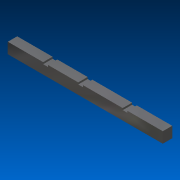
# Autodesk Inventor part: SPACER REAR B 1
Saved by Autodesk Inventor 2012 (Build 160160000, 160)
## iProperties
Created: 2012-07-06
Part Number: SPACER REAR B 1
Material: Default
Document SubType Name: Modeling
Designer: Hemant
Density: 1 g/cm^3
Author: Hemant
Autodesk Inventor part; units mm, degrees
ref_plane "YZ Plane" through (0, 0, 0) normal (1, 0, 0) x (0, 1, 0)
ref_plane "XZ Plane" through (0, 0, 0) normal (0, 1, 0) x (-1, 0, 0)
ref_plane "XY Plane" through (0, 0, 0) normal (0, 0, 1) x (1, 0, 0)
sketch "Sketch1" plane through (0, 0, 0) normal (0, 0, 1) x (1, 0, 0)
  line L0 (0, 0) -> (0, 58.2168)
  line L1 (0, 58.2168) -> (190.5, 58.2168)
  line L2 (190.5, 58.2168) -> (190.5, 48.6918)
  line L3 (190.5, 48.6918) -> (215.9, 48.6918)
  line L4 (215.9, 48.6918) -> (215.9, 58.2168)
  line L5 (215.9, 58.2168) -> (379.476, 58.2168)
  line L6 (379.476, 58.2168) -> (379.476, 48.6918)
  line L7 (379.476, 48.6918) -> (404.876, 48.6918)
  line L8 (404.876, 48.6918) -> (404.876, 58.2168)
  line L9 (404.876, 58.2168) -> (619.125, 58.2168)
  line L10 (619.125, 58.2168) -> (619.125, 48.6918)
  line L11 (619.125, 48.6918) -> (644.525, 48.6918)
  line L12 (644.525, 48.6918) -> (644.525, 58.2168)
  line L13 (644.525, 58.2168) -> (835.025, 58.2168)
  line L14 (835.025, 58.2168) -> (835.025, 0)
  line L15 (835.025, 0) -> (0, 0)
  dimension "d0" = 58.2168
  dimension "d1" = 835.025
  dimension "d2" = 190.5
  dimension "d3" = 25.4
  dimension "d4" = 25.4
  dimension "d5" = 25.4
  dimension "d6" = 9.525
  dimension "d7" = 190.5
  dimension "d8" = 163.576
  constraints: 32 end point, 11 parallel, 8 collinear, 1 perpendicular, 1 vertical
  measures "d0" distance between parallel lines of L15 L1
  measures "d1" distance between parallel lines of L14 L0
  measures "d2" distance from line of L2.end L0
  measures "d3" distance between parallel lines of L4 L2
  measures "d4" distance between parallel lines of L12 L10
  measures "d5" distance between parallel lines of L6 L8
  measures "d6" distance between parallel lines of L3 L1
  measures "d7" distance between parallel lines of L14 L12
  measures "d8" distance between parallel lines of L6 L4
extrude "Extrusion1" add sketch "Sketch1" along normal blind 50.8
body "Solid1"
